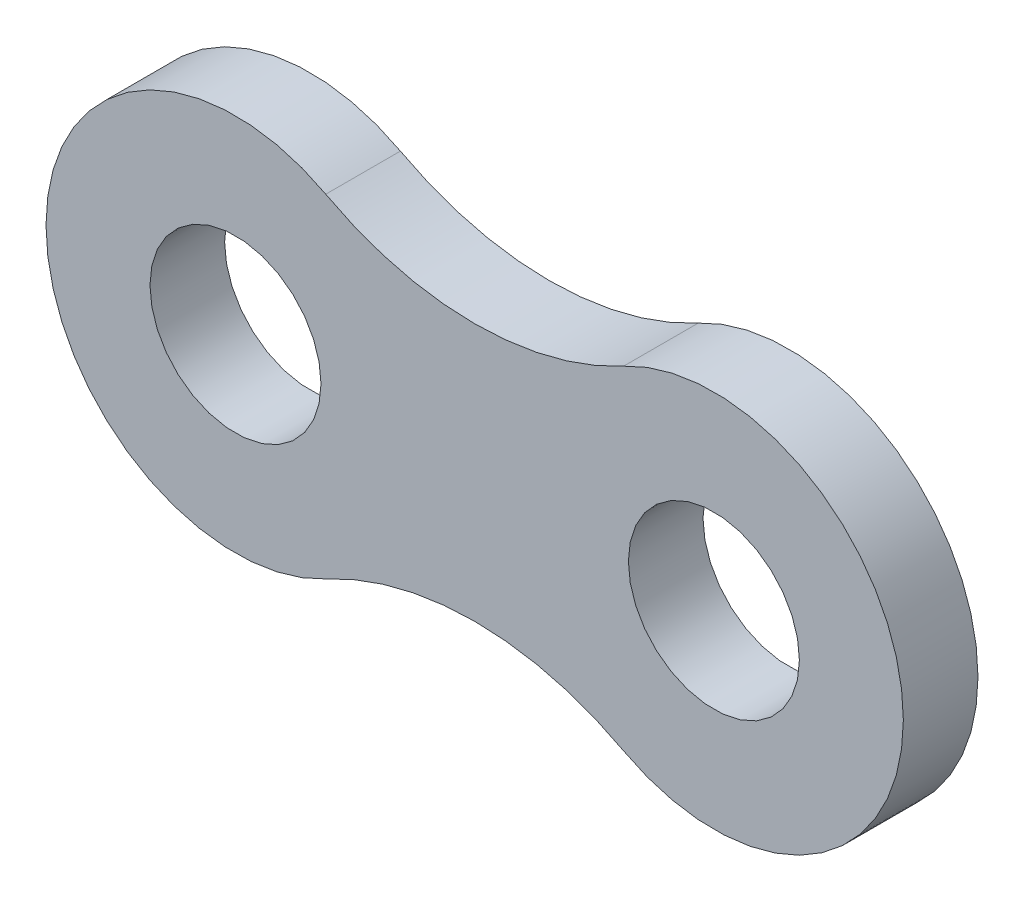
# Autodesk Inventor part: Chain Link
Saved by Autodesk Inventor 2017 (Build 210142000, 142)
## iProperties
Created: 2018-01-27
Part Number: Chain Link
Material: Generic
Document SubType Name: Modeling
Designer: 764368
Density: 1 g/cm^3
Appearance: Default
Author: 764368
Autodesk Inventor part; units mm, degrees
ref_plane "YZ Plane" through (0, 0, 0) normal (1, 0, 0) x (0, 1, 0)
ref_plane "XZ Plane" through (0, 0, 0) normal (0, 1, 0) x (-1, 0, 0)
ref_plane "XY Plane" through (0, 0, 0) normal (0, 0, 1) x (1, 0, 0)
sketch "Sketch1" plane through (0, 0, 0) normal (0, 0, 1) x (1, 0, 0)
  arc A0 (-11.9712, 1.9221) -> (-8.0178, 1.9221) centre (-9.9945, 5.5697) ccw projected
  arc A1 (-8.0178, -2.5002) -> (-8.0178, 1.9221) centre (-6.8195, -0.289) ccw projected
  arc A2 (-8.0178, -2.5002) -> (-11.9712, -2.5002) centre (-9.9945, -6.1478) ccw projected
  arc A3 (-11.9712, 1.9221) -> (-11.9712, -2.5002) centre (-13.1695, -0.289) ccw projected
  circle A4 centre (-13.1695, -0.289) radius 1.135 projected
  circle A5 centre (-6.8195, -0.289) radius 1.135 projected
  point P0 (0, 0)
extrude "Extrusion1" add sketch "Sketch1" along normal blind 0.9906
body "Solid1"
